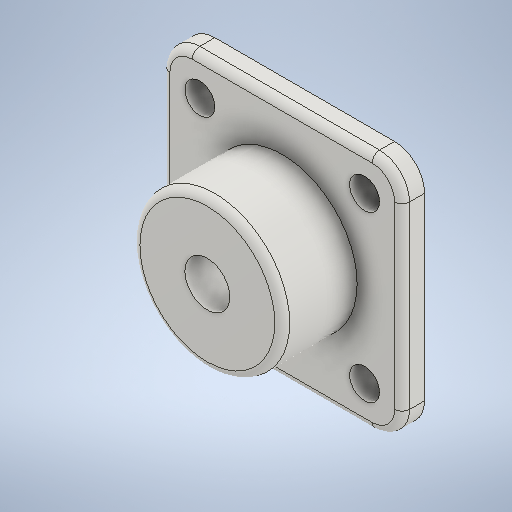
# Autodesk Inventor part: 12B VALVE BONNET
Saved by Autodesk Inventor 2025.2 (Build 292293000, 293)
## iProperties
Created: 2025-05-29
Part Number: 12B VALVE BONNET
Material: Steel AISI 1020 107 HR
Document SubType Name: Modeling
Designer: bless
Density: 7.87 g/cm^3
Appearance: Steel
Author: bless
Autodesk Inventor part; units mm, degrees
ref_plane "YZ Plane" through (0, 0, 0) normal (1, 0, 0) x (0, 1, 0)
ref_plane "XZ Plane" through (0, 0, 0) normal (0, 1, 0) x (-1, 0, 0)
ref_plane "XY Plane" through (0, 0, 0) normal (0, 0, 1) x (1, 0, 0)
sketch "Sketch1" plane through (0, 0, 0) normal (0, 0, 1) x (1, 0, 0)
  line L0 (-6, 8) -> (6, 8)
  line L1 (8, 6) -> (8, -6)
  line L2 (6, -8) -> (-6, -8)
  line L3 (-8, -6) -> (-8, 6)
  line L4 (-8, 8) -> (8, -8) construction
  line L5 (8, 8) -> (-8, -8) construction
  arc A0 (-6, 8) -> (-8, 6) centre (-6, 6) ccw
  arc A1 (-8, -6) -> (-6, -8) centre (-6, -6) ccw
  arc A2 (8, 6) -> (6, 8) centre (6, 6) ccw
  arc A3 (6, -8) -> (8, -6) centre (6, -6) ccw
  point P0 (0, 0)
  dimension "d0" = 16
  dimension "d1" = 16
  dimension "d2" = 2
  constraints: 12 end point, 8 point on circle, 8 point on line, 8 tangent, 4 centre point, 3 equal radius, 2 midpoint, 2 parallel, 1 horizontal, 1 perpendicular
  measures "d0" distance of L5.start L4.end
  measures "d1" distance of L4.start L5.start
  measures "d2" radius of A0
extrude "Extrusion1" add sketch "Sketch1" along normal blind 1.5
sketch "Sketch2" plane through (0, 0, 1.5) normal (0, 0, 1) x (1, 0, 0)
  circle A0 centre (0, 0) radius 5
  dimension "d5" = 10
  constraints: 1 centre point, 1 coincident
  measures "d5" diameter of A0
extrude "Extrusion2" add sketch "Sketch2" along normal blind 5
fillet "Fillet1" radius 0.5 9 edges at (-5, 0, 6.5) (-7.4142, 7.4142, 1.5) (-8, 0, 1.5) (-7.4142, -7.4142, 1.5) (0, -8, 1.5) (7.4142, -7.4142, 1.5) (8, 0, 1.5) (7.4142, 7.4142, 1.5) (0, 8, 1.5)
sketch "Sketch3" plane through (0, 0, 6.5) normal (0, 0, 1) x (1, 0, 0)
  circle A0 centre (0, 0) radius 4.5 projected
  circle A1 centre (0, 0) radius 1.5
  dimension "d9" = 3
  constraints: 1 centre point, 1 coincident
  measures "d9" diameter of A1
extrude "Extrusion3" cut sketch "Sketch3" against normal through all contours A1
sketch "Sketch4" plane through (0, 0, 0) normal (0, 0, -1) x (-1, 0, 0)
  circle A0 centre (0, 0) radius 1.5 projected
  circle A1 centre (0, 0) radius 4
  dimension "d12" = 8
  constraints: 1 centre point, 1 coincident
  measures "d12" diameter of A1
extrude "Extrusion4" cut sketch "Sketch4" against normal blind 2.5
sketch "Sketch5" plane through (0, 0, 0) normal (0, 0, -1) x (-1, 0, 0)
  line L0 (6, -8) -> (-6, -8) projected
  line L1 (8, 6) -> (8, -6) projected
  line L2 (-8, -6) -> (-8, 6) projected
  circle A0 centre (-5.5, 5.5) radius 1
  circle A1 centre (5.5, 5.5) radius 1
  circle A2 centre (5.5, -5.5) radius 1
  circle A3 centre (-5.5, -5.5) radius 1
  dimension "d15" = 2.5
  dimension "d16" = 2.5
  dimension "d17" = 11
  dimension "d18" = 2
  dimension "d19" = 2.5
  constraints: 4 centre point, 3 equal radius, 2 horizontal alignment, 2 vertical alignment
  measures "d15" distance from line of L0 A3.centre
  measures "d16" distance from line of L2 A3.centre
  measures "d17" distance of A2.centre A1.centre
  measures "d18" diameter of A3
  measures "d19" distance from line of L1 A1.centre
extrude "Extrusion5" cut sketch "Sketch5" against normal through all
body "Solid1"
